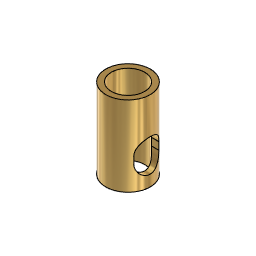
Extruder Gear Sleeve v3 (Autodesk Fusion 360 design; units mm, degrees)
Autodesk Fusion 360 part; units mm, degrees
note: some values were not read from the file. Set by a fixed rule: which sketch regions a step uses.
sketch "Sketch1" plane through (0, 0, 0) normal (0, 0, 1) x (1, 0, 0)
  circle A0 centre (0, 0) radius 3
  circle A1 centre (0, 0) radius 4
  dimension "d1" = 6
  dimension "d2" = 8
  constraint coincident A0.centre A1.centre
  measures "d1" diameter of A0
  measures "d2" diameter of A1
extrude "Extrude1" add sketch "Sketch1" along normal blind 14.4
sketch "Sketch2" plane through (0, 0, 0) normal (1, 0, 0) x (0, 1, 0)
  line L0 (0, 14.4) -> (0, 7.85)
  line L1 (0, 0) -> (0, 1.6)
  line L2 (0, 1.6) -> (0, 2)
  line L3 (0, 7.85) -> (0, 5.6)
  line L4 (0, 2) -> (0, 4.25)
  circle A0 centre (0, 4.25) radius 2.25
  circle A1 centre (0, 5.6) radius 2.25
  line L5 (0, 5.6) -> (-2.25, 5.6)
  line L6 (-2.25, 5.6) -> (-2.25, 4.25)
  line L7 (0, 5.6) -> (2.25, 5.6)
  line L8 (2.25, 5.6) -> (2.25, 4.25)
  dimension "d5" = 6.55
  dimension "d6" = 1.6
  dimension "d7" = 2.25
  dimension "d8" = 2.25
  constraint vertical L0
  constraint coincident L1.start origin
  constraint vertical L1
  constraint parallel L0 L3
  constraint parallel L2 L4
  constraint coincident L4.end A0.centre
  constraint coincident L2.end A0
  constraint coincident L3.end A1.centre
  constraint coincident L0.end A1
  constraint coincident A1 L5.end
  constraint perpendicular L3 L5
  constraint coincident A0 L6.end
  constraint tangent A0 L6
  constraint perpendicular L5 L6
  constraint coincident A1 L7.end
  constraint perpendicular L3 L7
  constraint coincident A0 L8.end
  constraint tangent A0 L8
  measures "d5" distance of L0.start L0.end
  measures "d6" distance of L1.start L1.end
  measures "d7" distance of L0.end L3.end
  measures "d8" distance of L2.end L4.end
extrude "Extrude2" cut sketch "Sketch2" along normal blind 9.083
named bodies: "Sleeve"
